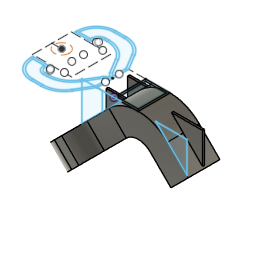
Fan Duct v2 (Autodesk Fusion 360 design; units mm, degrees)
Autodesk Fusion 360 part; units mm, degrees
sketch "Sketch1" plane through (0, 0, 0) normal (0, 0, 1) x (1, 0, 0)
  line L0 (0, 0) -> (12.5, 0)
  line L1 (12.5, 0) -> (12.5, 16.3)
  line L2 (12.5, 16.3) -> (0, 16.3)
  line L3 (0, 16.3) -> (0, 0)
  line L4 (1, 15.3) -> (11.5, 15.3)
  line L5 (11.5, 15.3) -> (11.5, 1)
  line L6 (11.5, 1) -> (1, 1)
  line L7 (1, 1) -> (1, 15.3)
  line L8 (-20, -1.85) -> (-40, -1.85) construction
  line L9 (-40, -1.85) -> (-40, 18.15) construction
  line L10 (-40, 18.15) -> (-20, 18.15) construction
  line L11 (-20, 18.15) -> (-20, -1.85) construction
  line L12 (-40, 8.15) -> (-35, 8.15) construction
  circle A0 centre (-35, 8.15) radius 3.85 construction
  line L13 (0, 16.3) -> (-8.75, 16.3) construction
  line L14 (0, 0) -> (-8.75, 0) construction
  line L15 (-8.75, 0) -> (-8.75, 16.3) construction
  line L16 (-39, 19) -> (-39, 20)
  line L17 (-29, 30) -> (-23.7815, 30)
  line L18 (-13.5016, 24.1905) -> (-8.75, 16.3)
  line L19 (-8.75, 8.15) -> (-9.022, 8.15)
  line L20 (-12.0204, 9.8444) -> (-16.5344, 17.3405)
  line L21 (-26.8144, 23.15) -> (-28.5, 23.15)
  line L22 (-31, 20.65) -> (-31, 19)
  arc A1 (-28.5, 23.15) -> (-31, 20.65) centre (-28.5, 20.65) ccw
  arc A2 (-16.5344, 17.3405) -> (-26.8144, 23.15) centre (-26.8144, 11.15) ccw
  arc A3 (-13.5016, 24.1905) -> (-23.7815, 30) centre (-23.7815, 18) ccw
  arc A4 (-29, 30) -> (-39, 20) centre (-29, 20) ccw
  arc A5 (-12.0204, 9.8444) -> (-9.022, 8.15) centre (-9.022, 11.65) ccw
  line L23 (-39, 19) -> (-31, 19)
  line L24 (-8.75, 16.3) -> (-8.75, 8.15)
  line L25 (-29, -13.7) -> (-23.7815, -13.7)
  arc A6 (-39, -3.7) -> (-29, -13.7) centre (-29, -3.7) ccw
  line L26 (-39, -2.7) -> (-39, -3.7)
  line L27 (-39, -2.7) -> (-31, -2.7)
  line L28 (-31, -4.35) -> (-31, -2.7)
  arc A7 (-31, -4.35) -> (-28.5, -6.85) centre (-28.5, -4.35) ccw
  line L29 (-26.8144, -6.85) -> (-28.5, -6.85)
  arc A8 (-26.8144, -6.85) -> (-16.5344, -1.0405) centre (-26.8144, 5.15) ccw
  line L30 (-12.0204, 6.4556) -> (-16.5344, -1.0405)
  arc A9 (-9.022, 8.15) -> (-12.0204, 6.4556) centre (-9.022, 4.65) ccw
  line L31 (-8.75, 8.15) -> (-9.022, 8.15)
  line L32 (-8.75, 0) -> (-8.75, 8.15)
  line L33 (-13.5016, -7.8905) -> (-8.75, 0)
  arc A10 (-23.7815, -13.7) -> (-13.5016, -7.8905) centre (-23.7815, -1.7) ccw
  line L34 (-32, 20.65) -> (-32, 20)
  line L35 (-38, 20) -> (-32, 20)
  arc A11 (-29, 29) -> (-38, 20) centre (-29, 20) ccw
  line L36 (-29, 29) -> (-23.7815, 29)
  arc A12 (-14.3582, 23.6746) -> (-23.7815, 29) centre (-23.7815, 18) ccw
  line L37 (-14.3582, 23.6746) -> (-9.75, 16.0221)
  line L38 (-9.75, 16.0221) -> (-9.75, 9.2583)
  arc A13 (-11.1637, 10.3603) -> (-9.75, 9.2583) centre (-9.022, 11.65) ccw
  line L39 (-11.1637, 10.3603) -> (-15.6778, 17.8564)
  arc A14 (-15.6778, 17.8564) -> (-26.8144, 24.15) centre (-26.8144, 11.15) ccw
  line L40 (-26.8144, 24.15) -> (-28.5, 24.15)
  arc A15 (-28.5, 24.15) -> (-32, 20.65) centre (-28.5, 20.65) ccw
  arc A16 (-9.75, 7.0417) -> (-11.1637, 5.9397) centre (-9.022, 4.65) ccw
  line L41 (-11.1637, 5.9397) -> (-15.6778, -1.5564)
  arc A17 (-26.8144, -7.85) -> (-15.6778, -1.5564) centre (-26.8144, 5.15) ccw
  line L42 (-26.8144, -7.85) -> (-28.5, -7.85)
  arc A18 (-32, -4.35) -> (-28.5, -7.85) centre (-28.5, -4.35) ccw
  line L43 (-32, -4.35) -> (-32, -3.7)
  line L44 (-38, -3.7) -> (-32, -3.7)
  arc A19 (-38, -3.7) -> (-29, -12.7) centre (-29, -3.7) ccw
  line L45 (-29, -12.7) -> (-23.7815, -12.7)
  arc A20 (-23.7815, -12.7) -> (-14.3582, -7.3746) centre (-23.7815, -1.7) ccw
  line L46 (-14.3582, -7.3746) -> (-9.75, 0.2779)
  line L47 (-9.75, 0.2779) -> (-9.75, 7.0417)
  line L48 (-8.75, 0) -> (-8.75, 1)
  dimension "d1" = 12.5
  dimension "d2" = 16.3
  dimension "d5" = 10.5
  dimension "d6" = 1
  dimension "d7" = 14.3
  dimension "d8" = 1
  dimension "d27" = 20
  dimension "d28" = 20
  dimension "d29" = 20
  dimension "d30" = 1.85
  dimension "d31" = 2.5
  dimension "d32" = 12
  dimension "d33" = 10
  dimension "d34" = 3.5
  dimension "d39" = 1
  dimension "d40" = -1
  constraint horizontal L0
  constraint vertical L1
  constraint horizontal L2
  constraint vertical L3
  constraint coincident L0.start L3.end
  constraint horizontal L4
  constraint vertical L5
  constraint horizontal L6
  constraint vertical L7
  constraint horizontal L8
  constraint vertical L9
  constraint horizontal L10
  constraint vertical L11
  constraint midpoint L9 L12.start
  constraint perpendicular L9 L12
  constraint coincident L12.end A0.centre
  constraint perpendicular L3 L13
  constraint perpendicular L3 L14
  constraint perpendicular L13 L15
  constraint vertical L16
  constraint perpendicular L16 L17
  constraint midpoint L15 L19.start
  constraint perpendicular L15 L19
  constraint parallel L18 L20
  constraint perpendicular L15 L21
  constraint perpendicular L19 L22
  constraint tangent L21 A1
  constraint tangent L22 A1
  constraint tangent L20 A2
  constraint tangent L21 A2
  constraint tangent L17 A3
  constraint tangent L18 A3
  constraint equal A2 A3
  constraint tangent L16 A4
  constraint tangent L17 A4
  constraint tangent L19 A5
  constraint tangent L20 A5
  constraint perpendicular L22 L23
  constraint symmetric L12 L13.end L14.end
  constraint symmetric L12 L16.start L26.start
  constraint symmetric L12 L19.start L24.end
  constraint symmetric L12 L22.end L27.end
  constraint symmetric L12 L21.end A7.end
  constraint symmetric L12 L22.start L28.start
  constraint symmetric L12 A1 A7
  constraint symmetric L12 L20.end A8.end
  constraint symmetric L12 L21.start L29.start
  constraint symmetric L12 A2 A8
  constraint symmetric L12 L17.end L25.end
  constraint symmetric L12 L18.start L33.start
  constraint symmetric L12 A3 A10
  constraint symmetric L12 L16.end A6.start
  constraint symmetric L12 L17.start L25.start
  constraint symmetric L12 A4 A6
  constraint symmetric L12 L19.end A5.end
  constraint symmetric L12 L20.start L30.start
  constraint symmetric L12 A5 A9
  constraint coincident L32 L48.end
  constraint coincident L15 L48.end
  measures "d1" distance of L0.start L0.end
  measures "d2" distance of L0.start L2.end
  measures "d5" distance of L5 L7
  measures "d6" distance of L1 L5
  measures "d7" distance of L4 L6
  measures "d8" distance of L2 L4
  measures "d27" distance of L9.end L10.end
  measures "d28" distance of L8.end L9.end
  measures "d29" distance of L3 L11
  measures "d30" vertical distance of L2.end L10.end
  measures "d31" radius of A1
  measures "d32" radius of A2
  measures "d33" radius of A4
  measures "d34" radius of A5
sketch "Sketch2" plane through (0, 0, 0) normal (0, 1, 0) x (1, 0, 0)
  line L0 (6.25, 0) -> (6.25, -15)
  line L1 (0, 0) -> (12.5, 0)
  arc A0 (-8.75, -30) -> (6.25, -15) centre (-8.75, -15) ccw
  point P0 (6.25, -30)
  dimension "d9" = 6.25
  dimension "d10" = 30
  dimension "d12" = 15
  dimension "d25" = 15
  dimension "d26" = 15
  constraint vertical L0
  constraint midpoint L0.start L1
  constraint coincident P0 L0
  constraint tangent L0 A0
  measures "d9" distance of L0 L1.start
  measures "d10" distance of P0 L1
  measures "d12" radius of A0
  measures "d25" vertical distance of L0.end A0.start
  measures "d26" distance of L0.end A0.centre
sweep "Sweep2" add profiles "Sketch1" path "Sketch2" along L0 A0 section 1 contours L0 L1 L2 L3 makes body 1
extrude "Extrude1" add sketch "Sketch1" along normal blind 1 from surface at 23.75 separate body contours L16 L17 L18 L19 L20 L21 L22 A1 A2 A3 A4 A5 L23 L24 L31 | L19 L25 A6 L26 L27 L28 A7 L29 A8 L30 A9 L31 L32 L33 A10 L48 | L34 L35 A11 L36 A12 L37 L38 A13 L39 A14 L40 A15 | A16 L41 A17 L42 A18 L43 L44 A19 L45 A20 L46 L47 makes body 2
extrude "Extrude2" add sketch "Sketch1" along normal blind 10.5 from surface at 24.75 contours L16 L17 L18 L19 L20 L21 L22 A1 A2 A3 A4 A5 L23 L24 L31 | L19 L25 A6 L26 L27 L28 A7 L29 A8 L30 A9 L31 L32 L33 A10 L48 bodies 2
extrude "Extrude3" add sketch "Sketch1" along normal blind 1 from surface at 35.25 contours L16 L17 L18 L19 L20 L21 L22 A1 A2 A3 A4 A5 L23 L24 L31 | L19 L25 A6 L26 L27 L28 A7 L29 A8 L30 A9 L31 L32 L33 A10 L48 | L34 L35 A11 L36 A12 L37 L38 A13 L39 A14 L40 A15 | A16 L41 A17 L42 A18 L43 L44 A19 L45 A20 L46 L47 bodies 2
sketch "Sketch5" plane through (0, -2.7, 0) normal (0, 1, 0) x (-1, 0, 0)
  line L0 (31, 23.75) -> (39, 23.75)
  line L1 (39, 23.75) -> (39, 36.25)
  line L2 (39, 36.25) -> (31, 36.25)
  line L3 (31, 36.25) -> (31, 23.75)
  line L4 (32, 24.75) -> (38, 24.75)
  line L5 (38, 24.75) -> (38, 35.25)
  line L6 (38, 35.25) -> (32, 35.25)
  line L7 (32, 35.25) -> (32, 24.75)
  dimension "d47" = -1
extrude "Extrude4" cut sketch "Sketch5" against normal blind 1 contours L4 L5 L6 L7 bodies 2
sketch "Sketch6" plane through (0, 19, 0) normal (0, -1, 0) x (1, 0, 0)
  line L0 (-39, 23.75) -> (-31, 23.75)
  line L1 (-31, 23.75) -> (-31, 36.25)
  line L2 (-31, 36.25) -> (-39, 36.25)
  line L3 (-39, 36.25) -> (-39, 23.75)
  line L4 (-38, 24.75) -> (-32, 24.75)
  line L5 (-32, 24.75) -> (-32, 35.25)
  line L6 (-32, 35.25) -> (-38, 35.25)
  line L7 (-38, 35.25) -> (-38, 24.75)
  dimension "d50" = -1
extrude "Extrude5" cut sketch "Sketch6" against normal blind 1 contours L4 L5 L6 L7 bodies 2
sketch "Sketch7" plane through (-8.75, 0, 0) normal (1, 0, 0) x (0, 1, 0)
  line L0 (0, 23.75) -> (16.3, 23.75)
  line L1 (16.3, 23.75) -> (16.3, 36.25)
  line L2 (16.3, 36.25) -> (0, 36.25)
  line L3 (0, 36.25) -> (0, 23.75)
  line L4 (0, 36.25) -> (16.3, 36.25)
  line L5 (16.3, 36.25) -> (16.3, 23.75)
  line L6 (16.3, 23.75) -> (0, 23.75)
  line L7 (0, 23.75) -> (0, 36.25)
  line L8 (7.15, 35.25) -> (7.15, 24.75)
  line L9 (9.15, 35.25) -> (9.15, 24.75)
  line L10 (1, 24.75) -> (1, 35.25)
  line L11 (15.3, 35.25) -> (15.3, 24.75)
  line L12 (1, 35.25) -> (7.15, 35.25)
  line L13 (9.15, 35.25) -> (15.3, 35.25)
  line L14 (15.3, 24.75) -> (9.15, 24.75)
  line L15 (7.15, 24.75) -> (1, 24.75)
  constraint horizontal L4
  constraint vertical L5
  constraint horizontal L6
  constraint vertical L7
  constraint coincident L0.end L1.start
  constraint coincident L2.end L3.start
  constraint collinear L12 L13
  constraint collinear L14 L15
extrude "Extrude6" cut sketch "Sketch7" against normal blind 1 contours L8 L10 L12 L15 | L9 L11 L13 L14 bodies 2
move_body "Move1" bodies 1 2 to x (0.707107, 0, 0.707107) y (0, 1, 0) z (-0.707107, 0, 0.707107) at (29.257, 0, -25.6326)
sketch "Sketch8" plane through (0, 0, 0) normal (0, 1, 0) x (1, 0, 0)
  line L0 (37.5, 16) -> (21.5, 0)
  line L1 (21.5, 0) -> (37.5, 0)
  line L2 (37.5, 0) -> (37.5, 16)
  line L3 (-16.5, 20) -> (3.5, 0)
  line L4 (3.5, 0) -> (-16.5, 0)
  line L5 (-16.5, 0) -> (-16.5, 20)
  line L6 (-6, 9.5) -> (-6, 0)
  constraint horizontal L1
  constraint perpendicular L1 L2
  constraint horizontal L4
  constraint perpendicular L4 L5
  constraint coincident L3 L6.start
  constraint coincident L4 L6.end
  constraint perpendicular L4 L6
extrude "Extrude7" add 1 faces at (28.9034, 15.3, -18.9151) along direction (0, -1, 0) blind 2 from surface at 6.15 on bodies 1 bodies 1
fillet "Fillet1" radius 3 8 edges at (24.6608, 15.3, -19.6222) (12.4632, 15.3, -11.4632) (12.4632, 9.15, -11.4632) (24.6608, 9.15, -19.6222) (24.6608, 1, -19.6222) (12.4632, 1, -11.4632) (24.6608, 7.15, -19.6222) (12.4632, 7.15, -11.4632) on bodies 1
extrude "Extrude8" add sketch "Sketch8" along normal blind 1 from surface at 8 separate body contours L0 L1 L2 makes body 3
extrude "Extrude9" add sketch "Sketch8" along normal blind 1 from surface at 2 separate body contours L3 L4 L6 makes body 4
extrude "Extrude10" add sketch "Sketch8" along normal blind 1 from surface at 13 separate body contours L3 L4 L6 makes body 5
